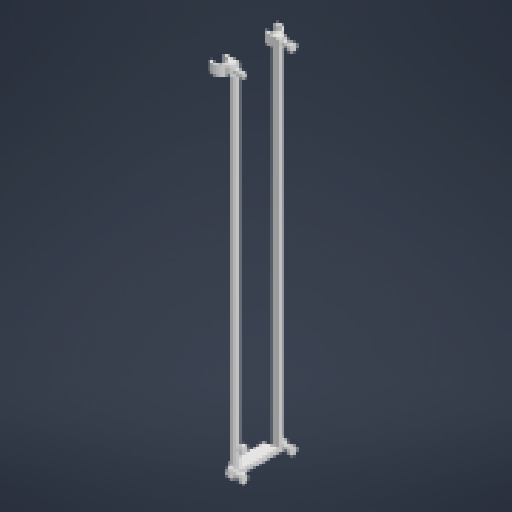
# Autodesk Inventor part: capFlipperConnectionPoint
Saved by Autodesk Inventor 2026 (Build 300175050, 175E)
## iProperties
Created: 2026-05-08
Part Number: capFlipperConnectionPoint
Material: Generic
Document SubType Name: Modeling
Designer: sniel
Density: 1 g/cm^3
Appearance: Default
Author: sniel
Autodesk Inventor part; units mm, degrees
ref_plane "YZ Plane" through (0, 0, 0) normal (1, 0, 0) x (0, 1, 0)
ref_plane "XZ Plane" through (0, 0, 0) normal (0, 1, 0) x (-1, 0, 0)
ref_plane "XY Plane" through (0, 0, 0) normal (0, 0, 1) x (1, 0, 0)
sketch "Sketch1" plane through (0, 0, 0) normal (0, 1, 0) x (-1, 0, 0)
  arc A0 (9.6258, 24.5172) -> (8.9916, 20.6504) centre (143.7343, 0.5373) ccw
  arc A1 (10.2149, 27.6058) -> (9.6258, 24.5172) centre (5, 27) ccw
  arc A2 (11.487, 33.26) -> (10.2149, 27.6058) centre (143.7343, 0.5373) ccw
  line L0 (11.487, 33.26) -> (6.6004, 34.3273)
  arc A3 (6.6004, 34.3273) -> (8.9916, 20.6504) centre (5, 27) ccw
  line L1 (6.6004, -33.2526) -> (11.487, -32.1853)
  arc A4 (10.2149, -26.5311) -> (11.487, -32.1853) centre (143.7343, 0.5373) ccw
  arc A5 (9.6258, -23.4425) -> (10.2149, -26.5311) centre (5, -25.9253) ccw
  arc A6 (8.9916, -19.5758) -> (9.6258, -23.4425) centre (143.7343, 0.5373) ccw
  arc A7 (8.9916, -19.5758) -> (6.6004, -33.2526) centre (5, -25.9253) ccw
  arc A8 (8.7273, 18.7917) -> (9.6258, -23.4425) centre (143.7343, 0.5373) ccw
  circle A9 centre (5, -25.9253) radius 5.25
  circle A10 centre (5, 27) radius 5.25
  circle A11 centre (5, 27) radius 7.5
  circle A12 centre (5, -25.9253) radius 7.5
  line L2 (9.6258, 24.5172) -> (10.2149, 27.6058)
  line L3 (9.9204, 26.0615) -> (7.9558, 26.4362)
  line L4 (9.6258, -23.4425) -> (10.2149, -26.5311)
  line L5 (9.9204, -24.9868) -> (7.9558, -25.3615)
  line L6 (6.6686, -18.6133) -> (9.3465, -32.6528)
  line L7 (9.243, 33.1844) -> (6.6686, 19.688)
  point P0 (-26.0547, 24.3051)
  point P1 (7.1497, -21.1356)
  point P2 (9.243, -32.1098)
  point P3 (8.7618, -29.5874)
  point P4 (7.1497, 22.2103)
  point P5 (8.7618, 30.6621)
  constraints: 20 point on circle, 16 end point, 10 centre point, 4 coincident, 3 midpoint, 2 point on line, 1 concentric, 1 perpendicular, 10 other
extrude "Extrusion1" add sketch "Sketch1" against normal blind 10 contours L7 A3 A11 A1 | A7 L6 A5 A12
sketch "Sketch2" plane through (0, 0, 0) normal (0, 1, 0) x (1, 0, 0)
  arc A0 (-8.7618, -30.6621) -> (-7.1497, -22.2103) centre (-5, -27) ccw
  line L0 (-8.7618, -30.6621) -> (-9.243, -33.1844)
  arc A1 (-9.243, -33.1844) -> (-6.6686, -19.688) centre (-5, -27) ccw
  line L1 (-6.6686, -19.688) -> (-7.1497, -22.2103)
  arc A2 (-6.6686, 18.6133) -> (-9.243, 32.1098) centre (-5, 25.9253) ccw
  line L2 (-9.243, 32.1098) -> (-8.7618, 29.5874)
  arc A3 (-7.1497, 21.1356) -> (-8.7618, 29.5874) centre (-5, 25.9253) ccw
  line L3 (-7.1497, 21.1356) -> (-6.6686, 18.6133)
  arc A4 (-6.6686, -19.688) -> (-6.6686, 18.6133) centre (-115.6445, -0.5373) ccw
  line L4 (-3.3314, 18.6133) -> (6.6686, 18.6133)
  line L5 (-3.3314, -19.688) -> (6.6686, -19.688)
  line L6 (6.6686, -19.688) -> (6.6686, -24.688)
  line L7 (6.6686, -24.688) -> (2.1347, -24.688)
  arc A5 (-9.243, -33.1844) -> (-6.6686, -19.688) centre (-5, -27) ccw projected
  line L8 (6.6686, 18.6133) -> (6.6686, 23.6133)
  line L9 (6.6686, 23.6133) -> (2.1347, 23.6133)
  point P0 (0, 0)
  dimension "d5" = 10
  dimension "d6" = 10
  dimension "d7" = 5
  dimension "d8" = 5
  constraints: 20 end point, 14 point on circle, 7 centre point, 3 perpendicular, 2 horizontal, 1 vertical
  measures "d5" distance of L4.start L4.end
  measures "d6" distance of L5.start L5.end
  measures "d7" distance of L5.end L6.end
  measures "d8" distance of L4.end L8.end
extrude "Extrusion2" add sketch "Sketch2" against normal blind 35 contours A1 L5 L6 L7 | A2 L9 L8 L4
sketch "Sketch3" plane through (6.6686, 0, 24.688) normal (1, 0, 0) x (0, 0, -1)
  line L0 (0, 0) -> (5, 0) projected
  line L1 (0, 0) -> (0, -35) projected
  line L2 (5, -35) -> (0, -35) projected
  line L3 (5, 0) -> (5, -35) projected
  line L4 (43.3013, 0) -> (48.3013, 0) projected
  line L5 (43.3013, 0) -> (43.3013, -35) projected
  line L6 (48.3013, -35) -> (43.3013, -35) projected
  line L7 (48.3013, 0) -> (48.3013, -35) projected
  line L8 (0, -35) -> (0, -40)
  line L9 (0, -40) -> (48.3013, -40)
  line L10 (48.3013, -40) -> (48.3013, -35)
  line L11 (43.3013, -35) -> (5, -35)
  line L12 (5, -35) -> (0, -35) projected
  circle A0 centre (0, -35) radius 5
  circle A1 centre (48.3013, -35) radius 5
  line L13 (0, 0) -> (0, -5)
  circle A2 centre (0, -5) radius 5
  circle A3 centre (48.3013, -5) radius 5
  point P0 (24.688, 0)
  point P1 (48.3013, -30)
  point P2 (0, -30)
  point P3 (48.3013, -10)
  point P4 (0, -10)
  dimension "d11" = 5
  constraints: 10 end point, 3 coincident, 3 perpendicular, 2 point on line, 1 vertical, 12 other
  measures "d11" distance of L1.end L8.end
extrude "Extrusion3" add sketch "Sketch3" against normal up to surface (4.5339 mm away) contours L1 A2 | A0 L8 L2 | L11 A1 L9 A0 | L1 L8 A0 | L6 L10 A1 | L7 A1 L10 | A3 L7 picked at (-0.3989, -8.2849) picked at (50.6435, -3.5972)
sketch "Sketch4" plane through (6.6686, 0, 24.688) normal (1, 0, 0) x (0, 0, -1)
  line L0 (0, 0) -> (5, 0) projected
  line L1 (0, -10) -> (0, -30) projected
  arc A0 (0, -30) -> (0, -40) centre (0, -35) ccw projected
  line L2 (0, -40) -> (48.3013, -40) projected
  arc A1 (48.3013, -40) -> (48.3013, -30) centre (48.3013, -35) ccw projected
  line L3 (48.3013, -10) -> (48.3013, -30) projected
  line L4 (43.3013, 0) -> (48.3013, 0) projected
  line L5 (43.3013, 0) -> (43.3013, -35) projected
  line L6 (43.3013, -35) -> (5, -35) projected
  line L7 (5, 0) -> (5, -35) projected
  circle A2 centre (0, -35) radius 2.5
  line L8 (48.3013, -35) -> (43.3013, -35) projected
  circle A3 centre (48.3013, -35) radius 2.5
  arc A4 (0, 0) -> (0, -10) centre (0, -5) ccw projected
  arc A5 (48.3013, -10) -> (48.3013, 0) centre (48.3013, -5) ccw projected
  circle A6 centre (0, -5) radius 2.5
  circle A7 centre (48.3013, -5) radius 2.5
  point P0 (24.688, 0)
  dimension "d14" = 5
  dimension "d15" = 5
  dimension "d22" = 5
  dimension "d23" = 5
  constraints: 4 centre point, 4 coincident
  measures "d14" diameter of A2
  measures "d15" diameter of A3
  measures "d22" diameter of A6
  measures "d23" diameter of A7
extrude "Extrusion4" add sketch "Sketch4" along normal blind 10 contours A2 | A3 | A6 | A7
sketch "Sketch5" plane through (16.6686, -35, 24.688) normal (1, 0, 0) x (0, 0, -1)
  circle A0 centre (0, 0) radius 2.5 projected
  circle A1 centre (48.3013, 0) radius 2.5 projected
  line L0 (5, 35) -> (5, 0) projected
  circle A2 centre (48.3013, 0) radius 4
  circle A3 centre (0, 0) radius 4
  circle A4 centre (0, 25) radius 4
  circle A5 centre (48.3013, 30) radius 2.5 projected
  circle A6 centre (48.3013, 30) radius 4
  point P0 (24.688, 35)
  dimension "d18" = 8
  dimension "d19" = 8
  dimension "d24" = 8
  dimension "d25" = 8
  constraints: 4 centre point, 3 coincident
  measures "d18" diameter of A2
  measures "d19" diameter of A3
  measures "d24" diameter of A4
  measures "d25" diameter of A6
extrude "Extrusion5" add sketch "Sketch5" against normal blind 3 contours A0 | A1 | A2 | A3 | A4 | A6
fillet "Fillet1" radius 1 2 edges at (-3.3314, -22.5, 19.688) (-3.3314, -22.5, -18.6133)
sketch "Sketch6" plane through (6.6686, -35, 19.688) normal (0, 1, 0) x (1, 0, 0)
  arc A0 (-15.3959, 0.8962) -> (-16.2944, 43.1305) centre (-150.4029, 19.1506) ccw
  circle A1 centre (-150.4029, 19.1506) radius 138.4029
  line L0 (-15.3959, 0.8962) -> (-15.1424, 2.8801)
  line L1 (-15.3959, 37.405) -> (-15.1424, 35.4212)
  line L2 (-4.5339, 0) -> (-4.5339, 38.3013) projected
  line L3 (-15.1424, 35.4212) -> (-4.5339, 38.3013)
  line L4 (-15.1424, 2.8801) -> (-4.5339, 0)
  point P0 (-6.6686, 19.688)
  point P1 (-13.0288, 35.995)
  point P2 (-13.0288, 2.3063)
  dimension "d27" = 2
  dimension "d28" = 2
  constraints: 8 end point, 5 point on circle, 2 centre point, 1 coincident, 4 other
  measures "d27" distance of L0.start L0.end
  measures "d28" distance of L1.start L1.end
extrude "Extrusion6" add sketch "Sketch6" against normal blind 5 contours A1 L3 L2 L4
body "Solid1"
